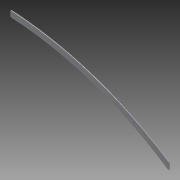
# Autodesk Inventor part: Ramp
Saved by Autodesk Inventor 2014 (Build 180170000, 170)
## iProperties
Created: 2014-01-20
Part Number: Ramp
Material: Aluminum 6061
Document SubType Name: Modeling
Designer: Andrew Toennies
Mass: 159.972 g
Surface Area: 419.88 cm^2
Volume: 59.0303 cm^3
Density: 2.71 g/cm^3
Appearance: Aluminum - Flat
Author: Andrew Toennies
Autodesk Inventor part; units mm, degrees
ref_plane "YZ Plane" through (0, 0, 0) normal (1, 0, 0) x (0, 1, 0)
ref_plane "XZ Plane" through (0, 0, 0) normal (0, 1, 0) x (-1, 0, 0)
ref_plane "XY Plane" through (0, 0, 0) normal (0, 0, 1) x (1, 0, 0)
sketch "Sketch1" plane through (0, 0, 0) normal (0, 0, 1) x (1, 0, 0)
  line L0 (342.9, 38.1) -> (342.9, 717.1861) construction
  line L1 (-606.2082, 101.6) -> (1077.8216, 101.6) construction
  line L2 (-65.7713, 38.1) -> (606.7605, 38.1) construction
  line L3 (685.8, 349.9428) -> (685.8, -276.2814) construction
  line L4 (-121.7677, -127) -> (863.1557, -127) construction
  arc A0 (684.3812, -126.0567) -> (3.3609, 101.407) centre (-77.2583, -1273.175) ccw
  arc A1 (680.8441, -154.2683) -> (2.9865, 75.9849) centre (-77.2583, -1273.175) ccw
  line L5 (0, 98.2375) -> (0, 79.1543)
  line L6 (685.8, -128.7018) -> (685.8, -151.6398)
  arc A2 (3.3609, 101.407) -> (0, 98.2375) centre (3.175, 98.2375) ccw
  arc A3 (0, 79.1543) -> (2.9865, 75.9849) centre (3.175, 79.1543) ccw
  arc A4 (680.8441, -154.2683) -> (685.8, -151.6398) centre (682.625, -151.6398) ccw
  arc A5 (685.8, -128.7018) -> (684.3812, -126.0567) centre (682.625, -128.7018) ccw
  point P0 (0, 0)
  point P1 (685.8, -127)
  point P2 (0, 101.6)
  point P3 (685.8, -157.6422)
  point P4 (0, 76.1592)
  dimension "d2" = 342.9
  dimension "d3" = 101.6
  dimension "d4" = 38.1
  dimension "d6" = 127
  dimension "d7" = 25.4
  dimension "d8" = 685.8
  dimension "d9" = 3.175
  constraints: 17 point on circle, 14 end point, 10 point on line, 8 tangent, 6 centre point, 3 equal radius, 3 vertical, 2 perpendicular, 1 collinear, 1 horizontal
  measures "d2" distance from line of point (0, 0) L0
  measures "d3" distance from line of point (0, 0) L1
  measures "d4" distance from line of point (0, 0) L2
  measures "d6" distance from line of point (0, 0) L4
  measures "d7" radial gap between concentric circles of A0 A1
  measures "d8" distance from line of point (0, 0) L3
  measures "d9" radius of A2
extrude "Extrusion1" add sketch "Sketch1" along normal blind 3.175
body "Solid1"
